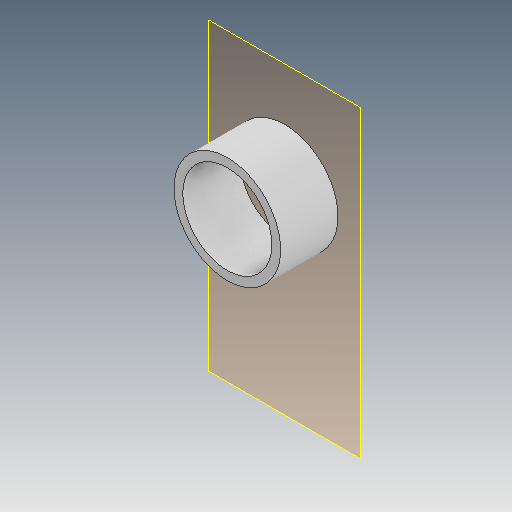
# Autodesk Inventor part: spacer for top of drivetrain
Saved by Autodesk Inventor 2020 (Build 240168000, 168)
## iProperties
Created: 2020-02-27
Part Number: spacer for top of drivetrain
Material: Generic
Document SubType Name: Modeling
Designer: jackm
Density: 1 g/cm^3
Appearance: Default
Author: jackm
Autodesk Inventor part; units mm, degrees
ref_plane "YZ Plane" through (0, 0, 0) normal (1, 0, 0) x (0, 1, 0)
ref_plane "XZ Plane" through (0, 0, 0) normal (0, 1, 0) x (-1, 0, 0)
ref_plane "XY Plane" through (0, 0, 0) normal (0, 0, 1) x (1, 0, 0)
ref_plane "Work Plane1" through (0, -0.0106, 0) normal (0, 0, 1) x (1, 0, 0)
sketch "Sketch1" plane through (0, -0.0106, 0) normal (0, 0, 1) x (1, 0, 0)
  arc A0 (-14.1209, 16.5181) -> (-15.151, 15.3922) centre (-16, 17.203) ccw construction
  circle A1 centre (-16, 17.203) radius 1.9304
  circle A2 centre (-16, 17.203) radius 2.3114
  point P0 (0, 0.0106)
  dimension "d0" = 3.8608
  dimension "d1" = 4.6228
  constraints: 2 centre point, 2 coincident
  measures "d0" diameter of A1
  measures "d1" diameter of A2
extrude "Extrusion1" add sketch "Sketch1" along normal blind 2.4892
body "Solid1"
